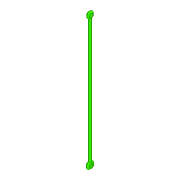
# Autodesk Inventor part: Delta Robot Arm Segment Two
Saved by Autodesk Inventor 2020 (Build 240168000, 168)
## iProperties
Created: 2021-03-06
Part Number: Delta Robot Arm Segment Two
Material: Generic
Document SubType Name: Modeling
Designer: Coy
Density: 1 g/cm^3
Appearance: Default(1)
Author: Coy
Autodesk Inventor part; units mm, degrees
ref_plane "YZ Plane" through (0, 0, 0) normal (1, 0, 0) x (0, 1, 0)
ref_plane "XZ Plane" through (0, 0, 0) normal (0, 1, 0) x (-1, 0, 0)
ref_plane "XY Plane" through (0, 0, 0) normal (0, 0, 1) x (1, 0, 0)
sketch "Sketch1" plane through (0, 0, 0) normal (1, 0, 0) x (0, 1, 0)
  circle A0 centre (0, 0) radius 2.5
  arc A1 (-4.0201, -2) -> (-4.0201, 2) centre (0, 0) ccw
  line L0 (0, 0) -> (-177.8, 0) construction
  circle A2 centre (-177.8, 0) radius 2.5
  arc A3 (-173.1955, 2) -> (-173.1955, -2) centre (-177.8, 0) ccw
  line L1 (-4.0201, 2) -> (-173.1955, 2)
  line L2 (-4.0201, -2) -> (-173.1955, -2)
  dimension "d0" = 5
  dimension "d1" = 1.9901
  dimension "d2" = 177.8
  dimension "d3" = 5
  dimension "d4" = 2.5201
  dimension "d9" = 4
  dimension "d10" = 2
  constraints: 6 end point, 4 centre point, 4 point on circle, 2 coincident, 2 parallel, 1 horizontal
  measures "d0" diameter of A0
  measures "d1" radial gap between concentric circles of A0 A1
  measures "d2" distance of L0.start L0.end
  measures "d3" diameter of A2
  measures "d4" radial gap between concentric circles of A2 A3
  measures "d9" distance between parallel lines of L2 L1
  measures "d10" distance between parallel lines of L0 L1
extrude "Extrusion1" add sketch "Sketch1" along normal blind 4
chamfer "Chamfer1" distance 1.6 angle 45 8 edges at (4, -88.6078, 2) (0, -88.6078, 2) (0, -88.6078, -2) (4, -88.6078, -2) (0, 4.4901, 0) (4, 4.4901, 0) (0, -182.8201, 0) (4, -182.8201, 0)
sketch "Sketch2" plane through (0, 0, 0) normal (0, 0, 1) x (1, 0, 0)
  line L0 (4, 2.5) -> (4, -2.5) projected
  line L1 (0, 2.5) -> (0, -2.5) projected
  line L2 (4, -175.3) -> (4, -180.3) projected
  line L3 (0, -175.3) -> (0, -180.3) projected
  line L4 (4, 2.5) -> (4, -2.5) construction
  line L5 (4, 0) -> (0, 0)
  line L6 (0, 2.5) -> (0, -2.5) construction
  line L7 (0, -175.3) -> (0, -180.3) construction
  line L8 (0, -177.8) -> (4, -177.8) construction
  line L9 (4, -175.3) -> (4, -180.3) construction
  circle A0 centre (2, 0) radius 3
  circle A1 centre (2, -177.8) radius 3
  line L10 (-1, -177.8) -> (5, -177.8)
  line L11 (5, 0) -> (-1, 0)
  dimension "d14" = 6
  dimension "d15" = 6
  constraints: 8 end point, 5 midpoint, 4 point on circle, 2 centre point, 1 parallel, 1 perpendicular, 1 point on line
  measures "d14" diameter of A0
  measures "d15" diameter of A1
revolve "Revolution1" cut sketch "Sketch2" angle 360 about axis through (-1, -177.8, 0) along (1, 0, 0) picked at (4.1409, -179.1351) picked at (2, -178.8) picked at (-0.1409, -179.1351) contours L10 A1 L2 | L2 A1 L3 L10 | L3 A1 L10
sketch "Sketch3" plane through (0, 0, 0) normal (0, 0, 1) x (1, 0, 0)
  line L0 (4, 2.5) -> (4, -2.5)
  line L1 (0, 2.5) -> (0, -2.5)
  line L2 (4, -175.3) -> (4, -180.3)
  line L3 (0, -175.3) -> (0, -180.3)
  line L4 (4, 2.5) -> (4, -2.5) construction
  line L5 (4, 0) -> (0, 0)
  line L6 (0, 2.5) -> (0, -2.5) construction
  line L7 (0, -175.3) -> (0, -180.3) construction
  line L8 (0, -177.8) -> (4, -177.8) construction
  line L9 (4, -175.3) -> (4, -180.3) construction
  circle A0 centre (2, 0) radius 3
  circle A1 centre (2, -177.8) radius 3
  line L10 (-1, -177.8) -> (5, -177.8)
  line L11 (5, 0) -> (-1, 0)
  dimension "d17" = 6
  dimension "d18" = 6
  constraints: 24 end point, 5 midpoint, 4 point on circle, 2 centre point, 1 parallel, 1 perpendicular, 1 point on line
  measures "d17" diameter of A0
  measures "d18" diameter of A1
revolve "Revolution2" cut sketch "Sketch3" angle 360 about axis through (5, 0, 0) along (-1, 0, 0) picked at (4.1409, 1.3351) picked at (2, 1) picked at (-0.1409, 1.3351) contours A0 L11 L0 | L0 L5 L1 A0 | L1 L11 A0
body "Solid1"
